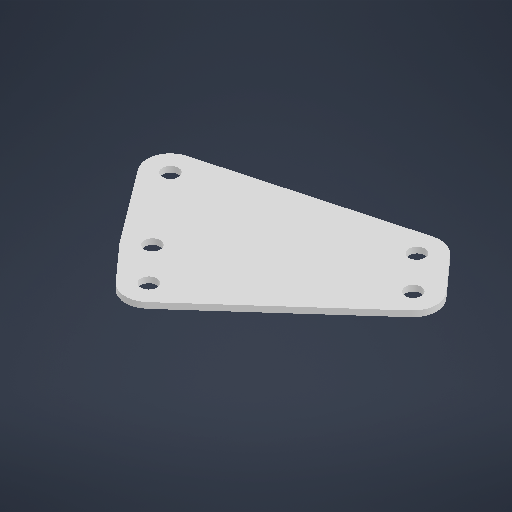
# Autodesk Inventor part: stackBrace
Saved by Autodesk Inventor 2025.2 (Build 292293000, 293)
## iProperties
Created: 2025-03-29
Part Number: stackBrace
Material: Generic
Document SubType Name: Modeling
Designer: Jahan
Density: 1 g/cm^3
Appearance: Default
Author: Jahan
Autodesk Inventor part; units mm, degrees
ref_plane "YZ Plane" through (0, 0, 0) normal (1, 0, 0) x (0, 1, 0)
ref_plane "XZ Plane" through (0, 0, 0) normal (0, 1, 0) x (-1, 0, 0)
ref_plane "XY Plane" through (0, 0, 0) normal (0, 0, 1) x (1, 0, 0)
sketch "Sketch1" plane through (0, 0, 0) normal (0, 1, 0) x (-1, 0, 0)
  circle A0 centre (-18.3582, -14.9546) radius 2.1844
  circle A1 centre (-26.8299, -5.4931) radius 2.1844
  circle A2 centre (34.045, -0.5216) radius 2.1844
  circle A3 centre (19.4876, 18.9331) radius 2.1844
  circle A4 centre (11.0156, 28.3943) radius 2.1844
  circle A5 centre (-18.3582, -14.9546) radius 6.35
  circle A6 centre (19.4876, 18.9331) radius 6.35
  circle A7 centre (34.045, -0.5216) radius 6.35
  circle A8 centre (11.0156, 28.3943) radius 6.35
  circle A9 centre (-26.8299, -5.4931) radius 6.35
  line L0 (6.7797, 33.125) -> (-31.0658, -0.7624)
  line L1 (15.7462, 32.6303) -> (24.2182, 23.1691)
  line L2 (-23.0889, -19.1904) -> (-31.5606, -9.729)
  line L3 (-16.672, -21.0766) -> (35.7311, -6.6437)
  line L4 (39.1292, 3.2827) -> (24.5718, 22.7374)
  point P0 (0, 0)
  dimension "d0" = 4.3688
  dimension "d1" = 4.3688
  dimension "d2" = 4.3688
  dimension "d3" = 12.7
  dimension "d4" = 12.7
  dimension "d5" = 12.7
  constraints: 12 tangent, 10 centre point, 10 end point, 10 point on circle, 5 coincident
  measures "d0" diameter of A2
  measures "d1" diameter of A3
  measures "d2" diameter of A4
  measures "d3" diameter of A5
  measures "d4" diameter of A6
  measures "d5" diameter of A7
extrude "Extrusion1" add sketch "Sketch1" along normal blind 1.5875
body "Solid1"
